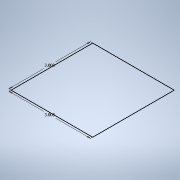
# Autodesk Inventor part: Block
Saved by Autodesk Inventor 2022 (Build 260153000, 153)
## iProperties
Created: 2022-03-02
Part Number: Block
Material: Generic
Document SubType Name: Modeling
Designer: Nathan Griffith
Density: 1 g/cm^3
Appearance: Default
Author: Nathan Griffith
Autodesk Inventor part; units mm, degrees
ref_plane "YZ Plane" through (0, 0, 0) normal (1, 0, 0) x (0, 1, 0)
ref_plane "XZ Plane" through (0, 0, 0) normal (0, 1, 0) x (-1, 0, 0)
ref_plane "XY Plane" through (0, 0, 0) normal (0, 0, 1) x (1, 0, 0)
sketch "Sketch1" plane through (0, 0, 0) normal (0, 1, 0) x (-1, 0, 0)
  line L0 (0, 0) -> (76.2, 0)
  line L1 (76.2, 0) -> (76.2, 76.2)
  line L2 (76.2, 76.2) -> (0, 76.2)
  line L3 (0, 76.2) -> (0, 0)
  dimension "d0" = 76.2
  dimension "d1" = 76.2
  constraints: 8 end point, 2 parallel, 1 horizontal, 1 perpendicular
  measures "d0" distance of L2.end L1.end
  measures "d1" distance of L1.end L0.end
extrude "Extrusion1" add sketch "Sketch1" along normal blind 2.54
sketch "Sketch2" plane through (0, 2.54, 0) normal (0, 1, 0) x (1, 0, 0)
  line L0 (-76.2, 0) -> (-76.2, -76.2) projected
  line L1 (-76.2, -76.2) -> (0, -76.2) projected
  line L2 (0, -76.2) -> (0, 0) projected
  line L3 (0, 0) -> (-76.2, 0) projected
  line L4 (-3.81, -3.81) -> (-3.81, -72.39)
  line L5 (-72.39, -3.81) -> (-54.39, -3.81)
  line L6 (-54.39, -3.81) -> (-54.39, -21.81)
  line L7 (-54.39, -21.81) -> (-72.39, -21.81)
  line L8 (-72.39, -21.81) -> (-72.39, -3.81)
  line L9 (-28.99, -3.81) -> (-28.99, -21.81)
  line L10 (-46.99, -3.81) -> (-28.99, -3.81)
  line L11 (-46.99, -21.81) -> (-46.99, -3.81)
  line L12 (-28.99, -21.81) -> (-46.99, -21.81)
  line L13 (-3.59, -3.81) -> (-3.59, -21.81)
  line L14 (-21.59, -3.81) -> (-3.59, -3.81)
  line L15 (-21.59, -21.81) -> (-21.59, -3.81)
  line L16 (-3.59, -21.81) -> (-21.59, -21.81)
  line L17 (-54.39, -29.21) -> (-54.39, -47.21)
  line L18 (-72.39, -29.21) -> (-54.39, -29.21)
  line L19 (-72.39, -47.21) -> (-72.39, -29.21)
  line L20 (-54.39, -47.21) -> (-72.39, -47.21)
  line L21 (-28.99, -29.21) -> (-28.99, -47.21)
  line L22 (-46.99, -29.21) -> (-28.99, -29.21)
  line L23 (-46.99, -47.21) -> (-46.99, -29.21)
  line L24 (-28.99, -47.21) -> (-46.99, -47.21)
  line L25 (-3.59, -29.21) -> (-3.59, -47.21)
  line L26 (-21.59, -29.21) -> (-3.59, -29.21)
  line L27 (-21.59, -47.21) -> (-21.59, -29.21)
  line L28 (-3.59, -47.21) -> (-21.59, -47.21)
  line L29 (-54.39, -54.61) -> (-54.39, -72.61)
  line L30 (-72.39, -54.61) -> (-54.39, -54.61)
  line L31 (-72.39, -72.61) -> (-72.39, -54.61)
  line L32 (-54.39, -72.61) -> (-72.39, -72.61)
  line L33 (-28.99, -54.61) -> (-28.99, -72.61)
  line L34 (-46.99, -54.61) -> (-28.99, -54.61)
  line L35 (-46.99, -72.61) -> (-46.99, -54.61)
  line L36 (-28.99, -72.61) -> (-46.99, -72.61)
  line L37 (-3.59, -54.61) -> (-3.59, -72.61)
  line L38 (-21.59, -54.61) -> (-3.59, -54.61)
  line L39 (-21.59, -72.61) -> (-21.59, -54.61)
  line L40 (-3.59, -72.61) -> (-21.59, -72.61)
  dimension "d4" = 3.81
  dimension "d5" = 18
  dimension "d6" = 18
  dimension "d9" = 25.4
  dimension "d12" = 25.4
  constraints: 74 end point, 2 horizontal, 2 parallel, 1 perpendicular, 1 vertical, 64 other
  measures "d4" distance between parallel lines of L2 L4
  measures "d5" distance of L6.end L7.end
  measures "d6" distance of L5.end L6.end
  measures "d9" distance of L5.end L9.start
  measures "d12" distance of L5.end L17.start
body "Solid1"
